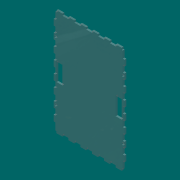
# Autodesk Inventor part: back
Saved by Autodesk Inventor 2016 (Build 200138000, 138)
## iProperties
Created: 2015-10-05
Part Number: back
Material: Polycarbonate, Clear
Document SubType Name: Modeling
Designer: Sawaiz
Density: 1.2 g/cm^3
Appearance: Polycarbonate - Clear
Author: Sawaiz
Autodesk Inventor part; units mm, degrees
ref_plane "YZ Plane" through (0, 0, 0) normal (1, 0, 0) x (0, 1, 0)
ref_plane "XZ Plane" through (0, 0, 0) normal (0, 1, 0) x (-1, 0, 0)
ref_plane "XY Plane" through (0, 0, 0) normal (0, 0, 1) x (1, 0, 0)
sketch "Sketch1" plane through (0, 0, 0) normal (0, 1, 0) x (-1, 0, 0)
  line L0 (60, -90) -> (-60, -90)
  line L1 (-60, -90) -> (-60, 90)
  line L2 (-60, 90) -> (60, 90)
  line L3 (60, 90) -> (60, -90)
  line L4 (60, -90) -> (-60, 90) construction
  line L5 (-60, -90) -> (60, 90) construction
  point P0 (0, 0)
  dimension "d0" = 120
  dimension "d1" = 180
  constraints: 12 end point, 2 midpoint, 2 parallel, 1 horizontal, 1 perpendicular
  measures "d0" distance of L1.end L2.end
  measures "d1" distance of L0.end L1.end
extrude "Extrusion1" add sketch "Sketch1" along normal blind 3.175
sketch "Sketch4" plane through (0, 0, 0) normal (0, -1, 0) x (1, 0, 0)
  line L0 (-60, -90) -> (60, -90) projected
  line L1 (60, -90) -> (60, 90) projected
  line L2 (60, 90) -> (-60, 90) projected
  line L3 (-60, 90) -> (-60, -90) projected
  line L4 (-60, 90) -> (60, 90) projected
  line L5 (-45, 90) -> (-35, 90)
  line L6 (-35, 90) -> (-35, 86.825)
  line L7 (-35, 86.825) -> (-45, 86.825)
  line L8 (-45, 86.825) -> (-45, 90)
  point P0 (0, 0)
  dimension "d25" = 10
  dimension "d26" = 15
  dimension "d27" = 3.175
  constraints: 8 end point, 2 parallel, 1 horizontal, 1 perpendicular, 1 point on line
  measures "d25" distance of L6.end L7.end
  measures "d26" distance between parallel lines of L3 L8
  measures "d27" distance of L7.end L5.start
extrude "Extrusion3" cut sketch "Sketch4" against normal through all contours L2 L6 L7 L8
pattern_linear "Rectangular Pattern1" count 6 spacing 20 along (1, 0, 0) of "Extrusion3"
sketch "Sketch7" plane through (0, 0, 0) normal (0, -1, 0) x (1, 0, 0)
  line L0 (55, 86.825) -> (55, 90) projected
  line L1 (55, 90) -> (45, 90) projected
  line L2 (45, 90) -> (45, 86.825) projected
  line L3 (45, 86.825) -> (35, 86.825) projected
  line L4 (35, 86.825) -> (35, 90) projected
  line L5 (35, 90) -> (25, 90) projected
  line L6 (25, 90) -> (25, 86.825) projected
  line L7 (25, 86.825) -> (15, 86.825) projected
  line L8 (15, 86.825) -> (15, 90) projected
  line L9 (15, 90) -> (5, 90) projected
  line L10 (5, 90) -> (5, 86.825) projected
  line L11 (5, 86.825) -> (-5, 86.825) projected
  line L12 (-5, 86.825) -> (-5, 90) projected
  line L13 (-5, 90) -> (-15, 90) projected
  line L14 (-15, 90) -> (-15, 86.825) projected
  line L15 (-15, 86.825) -> (-25, 86.825) projected
  line L16 (-25, 86.825) -> (-25, 90) projected
  line L17 (-25, 90) -> (-35, 90) projected
  line L18 (-35, 90) -> (-35, 86.825) projected
  line L19 (-35, 86.825) -> (-45, 86.825) projected
  line L20 (-45, 86.825) -> (-45, 90) projected
  line L21 (-45, 90) -> (-60, 90) projected
  line L22 (-60, 90) -> (-60, -90) projected
  line L23 (-60, -90) -> (60, -90) projected
  line L24 (60, -90) -> (60, 86.825) projected
  line L25 (60, 86.825) -> (55, 86.825) projected
  line L26 (-60, 90) -> (-55, 90)
  line L27 (-55, 90) -> (-55, 86.825)
  line L28 (-55, 86.825) -> (-60, 86.825)
  line L29 (-60, 86.825) -> (-60, 90)
  point P0 (0, 0)
  dimension "d50" = 10
  dimension "d51" = 3.175
  constraints: 8 end point, 2 parallel, 1 horizontal, 1 perpendicular
  measures "d50" distance between parallel lines of L20 L27
  measures "d51" distance between parallel lines of L21 L28
extrude "Extrusion5" cut sketch "Sketch7" against normal through all contours L22 L21 L27 L28
mirror "Mirror1" about plane through (0, 0, 0) normal (0, 0, 1) of "Extrusion3", "Rectangular Pattern1", "Extrusion5"
sketch "Sketch5" plane through (0, 0, 0) normal (0, -1, 0) x (1, 0, 0)
  line L0 (-35, -90) -> (-25, -90) projected
  line L1 (60, -86.825) -> (60, 86.825) projected
  line L2 (-45, 90) -> (-55, 90) projected
  line L3 (60, 86.825) -> (55, 86.825) projected
  line L4 (55, 86.825) -> (55, 90) projected
  line L5 (55, 90) -> (45, 90) projected
  line L6 (45, 90) -> (45, 86.825) projected
  line L7 (45, 86.825) -> (35, 86.825) projected
  line L8 (35, 86.825) -> (35, 90) projected
  line L9 (35, 90) -> (25, 90) projected
  line L10 (25, 90) -> (25, 86.825) projected
  line L11 (25, 86.825) -> (15, 86.825) projected
  line L12 (15, 86.825) -> (15, 90) projected
  line L13 (15, 90) -> (5, 90) projected
  line L14 (5, 90) -> (5, 86.825) projected
  line L15 (5, 86.825) -> (-5, 86.825) projected
  line L16 (-5, 86.825) -> (-5, 90) projected
  line L17 (-5, 90) -> (-15, 90) projected
  line L18 (-15, 90) -> (-15, 86.825) projected
  line L19 (-15, 86.825) -> (-25, 86.825) projected
  line L20 (-25, 86.825) -> (-25, 90) projected
  line L21 (-25, 90) -> (-35, 90) projected
  line L22 (-35, 90) -> (-35, 86.825) projected
  line L23 (-35, 86.825) -> (-45, 86.825) projected
  line L24 (-45, 86.825) -> (-45, 90) projected
  line L25 (-60, 86.825) -> (-60, -86.825) projected
  line L26 (-45, -90) -> (-45, -86.825) projected
  line L27 (-45, -86.825) -> (-35, -86.825) projected
  line L28 (-35, -86.825) -> (-35, -90) projected
  line L29 (-25, -90) -> (-25, -86.825) projected
  line L30 (-25, -86.825) -> (-15, -86.825) projected
  line L31 (-15, -86.825) -> (-15, -90) projected
  line L32 (-15, -90) -> (-5, -90) projected
  line L33 (-5, -90) -> (-5, -86.825) projected
  line L34 (-5, -86.825) -> (5, -86.825) projected
  line L35 (5, -86.825) -> (5, -90) projected
  line L36 (5, -90) -> (15, -90) projected
  line L37 (15, -90) -> (15, -86.825) projected
  line L38 (15, -86.825) -> (25, -86.825) projected
  line L39 (25, -86.825) -> (25, -90) projected
  line L40 (25, -90) -> (35, -90) projected
  line L41 (35, -90) -> (35, -86.825) projected
  line L42 (35, -86.825) -> (45, -86.825) projected
  line L43 (45, -86.825) -> (45, -90) projected
  line L44 (45, -90) -> (55, -90) projected
  line L45 (55, -90) -> (55, -86.825) projected
  line L46 (55, -86.825) -> (60, -86.825) projected
  line L47 (60, 90) -> (60, -90) projected
  line L48 (60, 85) -> (56.825, 85)
  line L49 (56.825, 85) -> (56.825, 75)
  line L50 (56.825, 75) -> (60, 75)
  line L51 (60, 75) -> (60, 85)
  line L52 (-55, -86.825) -> (-55, -90) projected
  line L53 (-55, -90) -> (-45, -90) projected
  line L54 (-55, 90) -> (-55, 86.825) projected
  line L55 (-55, 86.825) -> (-60, 86.825) projected
  line L56 (-60, -86.825) -> (-55, -86.825) projected
  point P0 (0, 0)
  dimension "d33" = 3.175
  dimension "d34" = 5
  dimension "d35" = 10
  constraints: 8 end point, 2 parallel, 1 horizontal, 1 perpendicular, 1 point on line
  measures "d33" distance of L48.start L48.end
  measures "d34" distance between parallel lines of L2 L48
  measures "d35" distance between parallel lines of L48 L50
extrude "Extrusion4" cut sketch "Sketch5" against normal through all contours L50 L49 L48 L1
pattern_linear "Rectangular Pattern2" count 9 spacing 20 along (0, 0, -1) of "Extrusion4"
sketch "Sketch8" plane through (0, 0, 0) normal (0, -1, 0) x (1, 0, 0)
  line L0 (56.825, -75) -> (60, -75) projected
  line L1 (60, -75) -> (60, -65) projected
  line L2 (60, -65) -> (56.825, -65) projected
  line L3 (56.825, -65) -> (56.825, -55) projected
  line L4 (56.825, -55) -> (60, -55) projected
  line L5 (60, -55) -> (60, -45) projected
  line L6 (60, -45) -> (56.825, -45) projected
  line L7 (56.825, -45) -> (56.825, -35) projected
  line L8 (56.825, -35) -> (60, -35) projected
  line L9 (60, -35) -> (60, -25) projected
  line L10 (60, -25) -> (56.825, -25) projected
  line L11 (56.825, -25) -> (56.825, -15) projected
  line L12 (56.825, -15) -> (60, -15) projected
  line L13 (60, -15) -> (60, -5) projected
  line L14 (60, -5) -> (56.825, -5) projected
  line L15 (56.825, -5) -> (56.825, 5) projected
  line L16 (56.825, 5) -> (60, 5) projected
  line L17 (60, 5) -> (60, 15) projected
  line L18 (60, 15) -> (56.825, 15) projected
  line L19 (56.825, 15) -> (56.825, 25) projected
  line L20 (56.825, 25) -> (60, 25) projected
  line L21 (60, 25) -> (60, 35) projected
  line L22 (60, 35) -> (56.825, 35) projected
  line L23 (56.825, 35) -> (56.825, 45) projected
  line L24 (56.825, 45) -> (60, 45) projected
  line L25 (60, 45) -> (60, 55) projected
  line L26 (60, 55) -> (56.825, 55) projected
  line L27 (56.825, 55) -> (56.825, 65) projected
  line L28 (56.825, 65) -> (60, 65) projected
  line L29 (60, 65) -> (60, 75) projected
  line L30 (60, 75) -> (56.825, 75) projected
  line L31 (56.825, 75) -> (56.825, 85) projected
  line L32 (56.825, 85) -> (60, 85) projected
  line L33 (60, 85) -> (60, 86.825) projected
  line L34 (60, 86.825) -> (55, 86.825) projected
  line L35 (55, 86.825) -> (55, 90) projected
  line L36 (55, 90) -> (45, 90) projected
  line L37 (45, 90) -> (45, 86.825) projected
  line L38 (45, 86.825) -> (35, 86.825) projected
  line L39 (35, 86.825) -> (35, 90) projected
  line L40 (35, 90) -> (25, 90) projected
  line L41 (25, 90) -> (25, 86.825) projected
  line L42 (25, 86.825) -> (15, 86.825) projected
  line L43 (15, 86.825) -> (15, 90) projected
  line L44 (15, 90) -> (5, 90) projected
  line L45 (5, 90) -> (5, 86.825) projected
  line L46 (5, 86.825) -> (-5, 86.825) projected
  line L47 (-5, 86.825) -> (-5, 90) projected
  line L48 (-5, 90) -> (-15, 90) projected
  line L49 (-15, 90) -> (-15, 86.825) projected
  line L50 (-15, 86.825) -> (-25, 86.825) projected
  line L51 (-25, 86.825) -> (-25, 90) projected
  line L52 (-25, 90) -> (-35, 90) projected
  line L53 (-35, 90) -> (-35, 86.825) projected
  line L54 (-35, 86.825) -> (-45, 86.825) projected
  line L55 (-45, 86.825) -> (-45, 90) projected
  line L56 (-45, 90) -> (-55, 90) projected
  line L57 (-55, 90) -> (-55, 86.825) projected
  line L58 (-55, 86.825) -> (-60, 86.825) projected
  line L59 (-60, 86.825) -> (-60, -86.825) projected
  line L60 (-60, -86.825) -> (-55, -86.825) projected
  line L61 (-55, -86.825) -> (-55, -90) projected
  line L62 (-55, -90) -> (-45, -90) projected
  line L63 (-45, -90) -> (-45, -86.825) projected
  line L64 (-45, -86.825) -> (-35, -86.825) projected
  line L65 (-35, -86.825) -> (-35, -90) projected
  line L66 (-35, -90) -> (-25, -90) projected
  line L67 (-25, -90) -> (-25, -86.825) projected
  line L68 (-25, -86.825) -> (-15, -86.825) projected
  line L69 (-15, -86.825) -> (-15, -90) projected
  line L70 (-15, -90) -> (-5, -90) projected
  line L71 (-5, -90) -> (-5, -86.825) projected
  line L72 (-5, -86.825) -> (5, -86.825) projected
  line L73 (5, -86.825) -> (5, -90) projected
  line L74 (5, -90) -> (15, -90) projected
  line L75 (15, -90) -> (15, -86.825) projected
  line L76 (15, -86.825) -> (25, -86.825) projected
  line L77 (25, -86.825) -> (25, -90) projected
  line L78 (25, -90) -> (35, -90) projected
  line L79 (35, -90) -> (35, -86.825) projected
  line L80 (35, -86.825) -> (45, -86.825) projected
  line L81 (45, -86.825) -> (45, -90) projected
  line L82 (45, -90) -> (55, -90) projected
  line L83 (55, -90) -> (55, -86.825) projected
  line L84 (55, -86.825) -> (60, -86.825) projected
  line L85 (60, -86.825) -> (60, -85) projected
  line L86 (60, -85) -> (56.825, -85) projected
  line L87 (56.825, -85) -> (56.825, -75) projected
  line L88 (56.825, 85) -> (60, 85)
  line L89 (60, 85) -> (60, 86.825)
  line L90 (60, 86.825) -> (56.825, 86.825)
  line L91 (56.825, 86.825) -> (56.825, 85)
  line L92 (56.825, -85) -> (60, -85)
  line L93 (60, -85) -> (60, -86.825)
  line L94 (60, -86.825) -> (56.825, -86.825)
  line L95 (56.825, -86.825) -> (56.825, -85)
  point P0 (0, 0)
  constraints: 16 end point, 4 parallel, 2 horizontal, 2 perpendicular
extrude "Extrusion6" cut sketch "Sketch8" against normal through all contours L86 L85 L84 L95 | L91 L34 L33 L32
mirror "Mirror2" about plane through (0, 0, 0) normal (1, 0, 0) of "Extrusion4", "Rectangular Pattern2", "Extrusion6"
sketch "Sketch6" plane through (0, 3.175, 0) normal (0, 1, 0) x (1, 0, 0)
  point P0 (0, 0)
  point P1 (56.825, -50)
  dimension "d41" = 50
  dimension "d42" = 56.825
  measures "d41" vertical distance of point (56.825, -50) point (0, 0)
  measures "d42" horizontal distance of point (0, 0) point (56.825, -50)
hole "Hole2" at (56.825, 3.175, 50) direction (0, -1, 0) diameter 3.4 end through all clearance for "Flat Head Machine Screw" size "M3" standard "Ansi Metric M Profile"
mirror "Mirror3" about plane through (0, 0, 0) normal (0, 0, 1) of "Hole2"
mirror "Mirror4" about plane through (0, 0, 0) normal (1, 0, 0) of "Hole2", "Mirror3"
sketch "Sketch9" plane through (0, 3.175, 0) normal (0, 1, 0) x (1, 0, 0)
  line L0 (45, -15) -> (55, -15)
  line L1 (55, -15) -> (55, 15)
  line L2 (55, 15) -> (45, 15)
  line L3 (45, 15) -> (45, -15)
  point P0 (0, 0)
  dimension "d56" = 30
  dimension "d57" = 10
  dimension "d58" = 45
  dimension "d62" = 15
  constraints: 8 end point, 2 parallel, 1 horizontal, 1 perpendicular
  measures "d56" distance of L2.end L0.start
  measures "d57" distance of L0.start L0.end
  measures "d58" distance from line of point (0, 0) L3
  measures "d62" distance from line of point (0, 0) L0
extrude "Extrusion7" cut sketch "Sketch9" against normal through all
mirror "Mirror5" about plane through (0, 0, 0) normal (1, 0, 0) of "Extrusion7"
sketch "Sketch3" plane through (0, 0, 0) normal (0, -1, 0) x (1, 0, 0)
  line L0 (43.8, 65) -> (43.8, -65) projected
  line L1 (43.8, -65) -> (-43.8, -65) projected
  line L2 (-43.8, -65) -> (-43.8, 65) projected
  line L3 (-43.8, 65) -> (43.8, 65) projected
  line L4 (-60, -90) -> (60, -90) projected
  line L5 (60, -90) -> (60, 90) projected
  line L6 (60, 90) -> (-60, 90) projected
  line L7 (-60, 90) -> (-60, -90) projected
  line L8 (58.5014, 54) -> (58.5014, 18)
  line L9 (58.5014, 18) -> (-58.5014, 18)
  line L10 (-58.5014, 18) -> (-58.5014, 54)
  line L11 (-20, 88.5014) -> (-20, -88.5014)
  line L12 (-20, -88.5014) -> (20, -88.5014)
  line L13 (-43.8, 65) -> (-43.8, -65) projected
  line L14 (20, -88.5014) -> (20, 88.5014)
  line L15 (58.5014, -54) -> (58.5014, -18)
  line L16 (58.5014, -18) -> (-58.5014, -18)
  line L17 (-43.8, 65) -> (43.8, 65) projected
  line L18 (43.8, -65) -> (-43.8, -65) projected
  line L19 (-58.5014, -18) -> (-58.5014, 18)
  line L20 (-58.5014, -54) -> (-58.5014, -18)
  line L21 (58.5014, -18) -> (58.5014, 18)
  line L22 (-58.5014, -54) -> (58.5014, -54)
  line L23 (-58.5014, 54) -> (58.5014, 54)
  line L24 (-20, 88.5014) -> (20, 88.5014)
  point P0 (0, 0)
  dimension "d9" = 1.5875
  dimension "d10" = 1.5875
  dimension "d11" = 1.5875
  dimension "d12" = 1.5875
  dimension "d20" = 40
  dimension "d21" = 40
  dimension "d22" = 36
  dimension "d24" = 36
  constraints: 29 end point, 5 vertical, 3 collinear, 3 horizontal, 3 parallel, 2 perpendicular
  measures "d20" distance from line of L7 L11.start
  measures "d21" distance of L11.start L14.end
  measures "d22" distance from line of L4 L20.start
  measures "d24" distance of L20.start L16.end
equation "\"d0\" = width"
equation "\"d1\" = height"
equation "\"d2\" = materialThickness"
equation "\"d25\" = notchWidth"
equation "\"d26\" = 1.5 * notchWidth"
equation "\"d27\" = materialThickness"
equation "\"d32\" = 2 * notchWidth"
equation "\"d50\" = notchWidth"
equation "\"d51\" = materialThickness"
equation "\"d33\" = materialThickness"
equation "\"d34\" = 0.5 * notchWidth"
equation "\"d35\" = notchWidth"
equation "\"d40\" = 2 * notchWidth"
equation "\"d41\" = 0.25 * height + 0.5 * notchWidth"
equation "\"d42\" = 0.5 * width - materialThickness"
equation "\"d9\" = 0.5 * materialThickness"
equation "\"d10\" = 0.5 * materialThickness"
equation "\"d11\" = 0.5 * materialThickness"
equation "\"d12\" = 0.5 * materialThickness"
equation "\"d20\" = 0.333333 * width"
equation "\"d21\" = 0.333333 * width"
equation "\"d22\" = 0.2 * height"
equation "\"d24\" = 0.2 * height"
equation "\"height\" = 180"
equation "\"width\" = 120"
equation "\"materialThickness\" = 3.175"
equation "\"laserKerf\" = 0.1"
equation "\"cardPinDiameter\" = 3"
equation "\"cardThickness\" = 0.76"
equation "\"cardFillet\" = 2.88"
equation "\"cardHeight\" = 53.98"
equation "\"cardSelected\" = 1"
equation "\"cardWidth\" = 85.6"
equation "\"centeralShaftDiameter\" = 8"
equation "\"cardClearence\" = 0.5"
equation "\"bearingOd\" = 22"
equation "\"bearingWidth\" = 8"
equation "\"axleHeight\" = 95"
equation "\"nutTrapClearence\" = 2"
equation "\"nutTrapwidth\" = 5.5"
equation "\"nutTrapDepth\" = 2.5"
equation "\"magnetDiameter\" = 6"
equation "\"magnetLength\" = 3"
equation "\"magnetProtusion\" = 0.25"
equation "\"notchWidth\" = 10"
equation "\"spoolThickness\" = 5.588"
body "Solid1"
